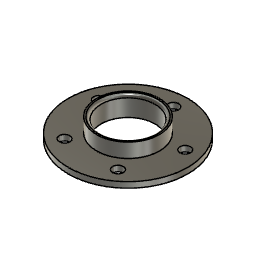
FinalFlange (Autodesk Fusion 360 design; units mm, degrees)
Autodesk Fusion 360 part; units mm, degrees
sketch "Sketch1" plane through (0, 0, 0) normal (0, 0, 1) x (1, 0, 0)
  circle A0 centre (0, 0) radius 28.067
  circle A1 centre (0, 0) radius 24.13
  circle A2 centre (0, 0) radius 53.467
  circle A3 centre (0, 40.64) radius 4.7625
  circle A4 centre (-38.6509, 12.5585) radius 4.7625
  circle A5 centre (-23.8876, -32.8785) radius 4.7625
  circle A6 centre (23.8876, -32.8785) radius 4.7625
  circle A7 centre (38.6509, 12.5585) radius 4.7625
  dimension "d1" = 56.134
  dimension "d2" = 48.26
  dimension "d3" = 106.934
  dimension "d4" = 9.525
  dimension "d6" = 360
  constraint coincident A0.centre A1.centre
  constraint concentric A0 A2
  measures "d1" diameter of A0
  measures "d2" diameter of A1
  measures "d3" diameter of A2
  measures "d4" diameter of A3
extrude "Extrude1" add sketch "Sketch1" against normal blind 5.08 contours A2
move_body "Move1" bodies 1 to x (1, 0, 0) y (0, 1, 0) z (0, 0, 1) at (0, 0, 5.08)
extrude "Extrude2" add sketch "Sketch1" along normal blind 17.78 contours A0
fillet "Fillet1" radius 2.54 1 edges at (-22.4971, 8.7258, 17.78)
